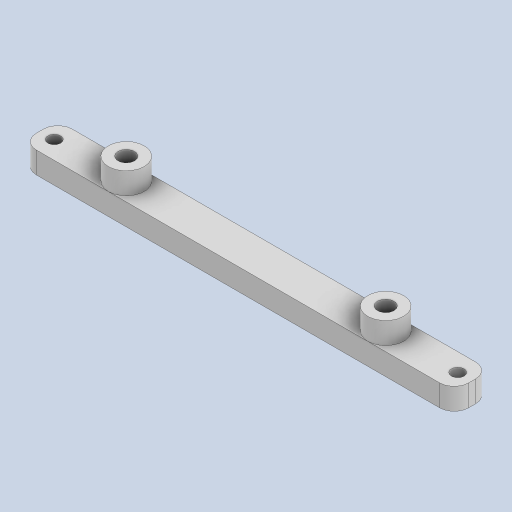
# Autodesk Inventor part: Busbar Base
Saved by Autodesk Inventor 2023 (Build 270158000, 158)
## iProperties
Created: 2023-03-08
Part Number: Busbar Base
Material: Generic
Document SubType Name: Modeling
Designer: cheng
Density: 1 g/cm^3
Appearance: Default
Author: cheng
Autodesk Inventor part; units mm, degrees
ref_plane "YZ Plane" through (0, 0, 0) normal (1, 0, 0) x (0, 1, 0)
ref_plane "XZ Plane" through (0, 0, 0) normal (0, 1, 0) x (-1, 0, 0)
ref_plane "XY Plane" through (0, 0, 0) normal (0, 0, 1) x (1, 0, 0)
sketch "Sketch1" plane through (0, 0, 0) normal (0, 1, 0) x (-1, 0, 0)
  line L0 (30, -2.5) -> (-30, -2.5)
  line L1 (-30, -2.5) -> (-30, 2.5)
  line L2 (-30, 2.5) -> (30, 2.5)
  line L3 (30, 2.5) -> (30, -2.5)
  line L4 (30, -2.5) -> (-30, 2.5) construction
  line L5 (-30, -2.5) -> (30, 2.5) construction
  point P0 (0, 0)
  dimension "d0" = 60
  dimension "d1" = 5
  constraints: 12 end point, 2 midpoint, 2 parallel, 1 horizontal, 1 perpendicular
  measures "d0" distance of L0.start L0.end
  measures "d1" distance between parallel lines of L2 L0
extrude "Extrusion1" add sketch "Sketch1" along normal blind 3
sketch "Sketch2" plane through (0, 3, 0) normal (0, 1, 0) x (1, 0, 0)
  line L0 (-30, -2.5) -> (30, -2.5) projected
  line L1 (30, -2.5) -> (30, 2.5) projected
  line L2 (30, 2.5) -> (-30, 2.5) projected
  line L3 (-30, 2.5) -> (-30, -2.5) projected
  line L4 (-30, 2.5) -> (30, -2.5) construction
  line L5 (30, 2.5) -> (-30, -2.5) construction
  line L6 (-30, 0) -> (30, 0) construction
  line L7 (0, 2.5) -> (0, -2.5) construction
  circle A0 centre (-18, 0) radius 2.5
  circle A1 centre (18, 0) radius 2.5
  point P0 (0, 0)
  dimension "d4" = 5
  dimension "d5" = 18
  constraints: 8 end point, 4 midpoint, 2 centre point, 1 point on line, 1 symmetric about line, 1 other
  measures "d4" diameter of A0
  measures "d5" distance from line of L7 A0.centre
extrude "Extrusion2" add sketch "Sketch2" along normal blind 3 contours A0 | A1
sketch "Sketch3" plane through (-18, 6, 0) normal (0, 1, 0) x (1, 0, 0)
  circle A0 centre (0, 0) radius 2.5 projected
  circle A1 centre (36, 0) radius 2.5 projected
  point P0 (18, 0)
  constraints: 2 coincident
hole "Hole1" at (-18, 6, 0) at (18, 6, 0) direction (0, -1, 0) diameter 2.3 end through all
fillet "Fillet1" radius 2 4 edges at (-30, 1.5, -2.5) (-30, 1.5, 2.5) (30, 1.5, -2.5) (30, 1.5, 2.5)
sketch "Sketch4" plane through (0, 3, 0) normal (0, 1, 0) x (1, 0, 0)
  arc A0 (28, -2.5) -> (30, -0.5) centre (28, -0.5) ccw projected
  line L0 (30, -0.5) -> (30, 0.5) projected
  arc A1 (30, 0.5) -> (28, 2.5) centre (28, 0.5) ccw projected
  line L1 (28, 2.5) -> (18, 2.5) projected
  arc A2 (-28, 2.5) -> (-30, 0.5) centre (-28, 0.5) ccw projected
  line L2 (-30, 0.5) -> (-30, -0.5) projected
  arc A3 (-30, -0.5) -> (-28, -2.5) centre (-28, -0.5) ccw projected
  line L3 (-28, -2.5) -> (-18, -2.5) projected
  arc A4 (18, -2.5) -> (18, 2.5) centre (18, 0) ccw projected
  arc A5 (-18, -2.5) -> (-18, 2.5) centre (-18, 0) ccw projected
  line L4 (-30, 0) -> (30, 0) construction
  line L5 (-28, 0.5) -> (-28, -0.5) construction
  line L6 (28, 0.5) -> (28, -0.5) construction
  arc A6 (18, 2.5) -> (18, -2.5) centre (18, 0) ccw projected
  line L7 (18, 2.5) -> (-18, 2.5) projected
  line L8 (-18, -2.5) -> (18, -2.5) projected
  arc A7 (-18, 2.5) -> (-18, -2.5) centre (-18, 0) ccw projected
  line L9 (-18, 2.5) -> (-28, 2.5) projected
  line L10 (18, -2.5) -> (28, -2.5) projected
  point P0 (0, 0)
  point P1 (-28, 0)
  point P2 (28, 0)
  constraints: 6 end point, 4 midpoint, 2 vertical
hole "Hole2" at (-28, 3, 0) at (28, 3, 0) direction (0, -1, 0) diameter 1.778 end through all
body "Solid1"
